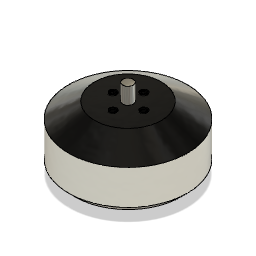
Tarot 630kv v2 (Autodesk Fusion 360 design; units mm, degrees)
Autodesk Fusion 360 part; units mm, degrees
sketch "Sketch1" plane through (0, 0, 0) normal (0, 1, 0) x (1, 0, 0)
  circle A0 centre (0, 0) radius 23.1
  dimension "d1" = 46.2
  constraint coincident A0.centre origin
  measures "d1" diameter of A0
extrude "Extrude1" add sketch "Sketch1" along normal blind 22
sketch "Sketch2" plane through (0, 22, 0) normal (0, 1, 0) x (-1, 0, 0)
  circle A0 centre (0, 0) radius 23.1
  circle A1 centre (0, 0) radius 2
  dimension "d4" = 4
  constraint coincident A0.centre A1.centre
  measures "d4" diameter of A1
extrude "Extrude2" add sketch "Sketch2" along normal blind 6.4 contours A1
sketch "Sketch3" plane through (0, 0, 0) normal (0, 0, 1) x (1, 0, 0)
  line L0 (23.1, 0) -> (23.1, 16)
  line L1 (-2, 22) -> (2, 22)
  line L2 (23.1, 22) -> (-23.1, 22)
  line L3 (0, 22) -> (13, 22)
  line L4 (13, 22) -> (23.1, 16)
  line L5 (13, 22) -> (23.1, 22)
  line L6 (23.1, 16) -> (23.1, 22)
  line L7 (23.1, 0) -> (23.1, 2.5)
  line L8 (23.1, 0) -> (20.6, 0)
  line L9 (20.6, 0) -> (23.1, 2.5)
  dimension "d7" = 16
  dimension "d8" = 13
  dimension "d10" = 2.5
  constraint vertical L0
  constraint midpoint L1 L3.start
  constraint parallel L2 L3
  constraint coincident L2.start L5.end
  constraint coincident L0 L7.end
  constraint perpendicular L0 L8
  measures "d7" distance of L0.start L0.end
  measures "d8" distance of L3.start L3.end
  measures "d10" distance of L0.start L8.end
revolve "Revolve2" cut sketch "Sketch3" angle 360 about axis through (0, 1.75, 0) along (0, 1, 0) contours L0 L7 L8 L9
revolve "Revolve1" cut sketch "Sketch3" angle 360 about axis through (0, 1.75, 0) along (0, 1, 0) contours L2 L4 L5 L6
sketch "Sketch4" plane through (0, 0, 0) normal (0, 1, 0) x (1, 0, 0)
  circle A0 centre (0, 0) radius 5
  circle A1 centre (0, 0) radius 4
  circle A2 centre (0, 0) radius 15.6
  circle A3 centre (15.6, 0) radius 1.5
  circle A4 centre (-7.8, 13.51) radius 1.5
  circle A5 centre (-7.8, -13.51) radius 1.5
  dimension "d12" = 10
  dimension "d13" = 31.2
  dimension "d14" = 3
  dimension "d16" = 360
  constraint coincident A0.centre A1.centre
  constraint concentric A0 A1
  constraint coincident A2 A3.centre
  measures "d12" diameter of A0
  measures "d13" diameter of A2
  measures "d14" diameter of A3
extrude "Extrude3" cut sketch "Sketch4" along normal blind 5 contours A2 A3 | A2 A3 | A2 A4 | A2 A4 | A2 A5 | A2 A5
extrude "Extrude4" add sketch "Sketch4" against normal blind 2.5 contours A1
thread "Thread1" "ISO Metric profile 3.0 M3x0.5 6H" major diameter 3.086 minor diameter 2.529 pitch 0.5 angle 60 modelled right hand crest width 0.1368 on face at (-6.3075, 1.6667, 13.6593) crest through (-6.5355, 0.125, 13.51) on face at (17.0925, 1.6667, 0.1494) crest through (16.8645, 0.125, 0) on face at (-6.3075, 3.3333, -13.6593) crest through (-6.5355, 0.125, -13.51)
sketch "Sketch5" plane through (0, 22, 0) normal (0, 1, 0) x (-1, 0, 0)
  circle A0 centre (0, 0) radius 13
  circle A1 centre (0, 0) radius 2
  circle A2 centre (0, 0) radius 6
  circle A3 centre (-6, 0) radius 1.5
  circle A4 centre (0, -6) radius 1.5
  circle A5 centre (6, 0) radius 1.5
  circle A6 centre (0, 6) radius 1.5
  dimension "d21" = 12
  dimension "d22" = 3
  dimension "d24" = 360
  constraint concentric A0 A2
  constraint coincident A2 A3.centre
  measures "d21" diameter of A2
  measures "d22" diameter of A3
extrude "Extrude5" cut sketch "Sketch5" against normal blind 4 contours A2 A5 | A2 A5 | A2 A6 | A2 A6 | A2 A4 | A2 A4 | A2 A3 | A2 A3
thread "Thread2" "ISO Metric profile 3.0 M3x0.5 6H" major diameter 3.086 minor diameter 2.529 pitch 0.5 angle 60 modelled right hand crest width 0.1368 on face at (-1.4925, 20.6667, -5.8506) crest through (-1.2645, 21.875, -6) on face at (-1.4925, 20.6667, 6.1494) crest through (-1.2645, 21.875, 6) on face at (-7.4981, 19.3333, -0.0748) crest through (-7.2645, 21.875, 0) on face at (4.5075, 20.6667, 0.1494) crest through (4.7355, 21.875, 0)
equation "d13 = ( 15.6 * 2 ) * 1 mm"
